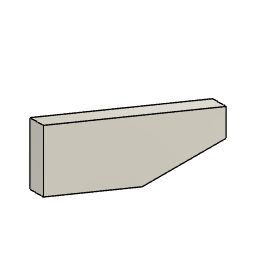
name_sign_support_left (Autodesk Fusion 360 design; units mm, degrees)
Autodesk Fusion 360 part; units mm, degrees
note: some values were not read from the file. Set by a fixed rule: which sketch regions a step uses.
sketch "Name Sign Support" plane through (0, 0, 0) normal (1, 0, 0) x (0, 1, 0) in component "Name Sign Support (1)"
  line L0 (-0.0158, 97.2466) -> (88.3556, 61.0028)
  line L1 (163.2949, 85.69) -> (-0.0158, 152.6686)
  line L2 (-0.0158, 152.6686) -> (-0.0158, 97.2466)
  line L3 (163.2949, 85.69) -> (163.2949, 61.0028)
  line L4 (88.3556, 61.0028) -> (163.2949, 61.0028)
  dimension "d18" = 67.7
  dimension "d9" = 55.422
  dimension "d2" = 176.512
  dimension "d3" = 95.515
  constraint vertical L2
  constraint parallel L2 L3
  constraint perpendicular L3 L4
  measures "d18" angle of L0 L3
  measures "d9" distance of L1.end L0.start
  measures "d2" distance of L1.start L1.end
  measures "d3" distance of L0.start L0.end
extrude "Extrude2" add sketch "Name Sign Support" along normal blind 12 in component "Name Sign Support (1)"
component "Name Sign Support Left" placed x (1, 0, 0) y (0, 1, 0) z (0, 0, 1) at (0, 0, 0)
component "Name Sign Support" placed x (1, 0, 0) y (0, 1, 0) z (0, 0, 1) at (0, 0, 0) in component "Name Sign Support Left"
component "Name Sign Support (1)" placed x (1, 0, 0) y (0, 1, 0) z (0, 0, 1) at (0, 0, 0) in component "Name Sign Support"
equation "d19 = pineThickness"
equation "pineThickness = 12 mm" comment "Thickness of the pine planks"
named bodies: "Name Sign Support"
